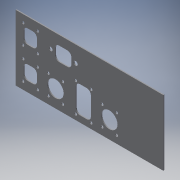
# Autodesk Inventor part: Plug-in Plate
Saved by Autodesk Inventor 2017 (Build 210142000, 142)
## iProperties
Created: 2017-03-05
Part Number: Plug-in Plate
Material: Generic
Document SubType Name: Modeling
Designer: coffmant
Density: 1 g/cm^3
Appearance: Default
Quantity: 1
Author: coffmant
Autodesk Inventor part; units mm, degrees
ref_plane "YZ Plane" through (0, 0, 0) normal (1, 0, 0) x (0, 1, 0)
ref_plane "XZ Plane" through (0, 0, 0) normal (0, 1, 0) x (-1, 0, 0)
ref_plane "XY Plane" through (0, 0, 0) normal (0, 0, 1) x (1, 0, 0)
sketch "Sketch1" plane through (0, 0, 0) normal (0, 0, 1) x (1, 0, 0)
  line L0 (0, 0) -> (228.6, 0)
  line L1 (228.6, 0) -> (228.6, -101.6)
  line L2 (228.6, -101.6) -> (0, -101.6)
  line L3 (0, -101.6) -> (0, 0)
  dimension "d0" = 101.6
  dimension "d1" = 228.6
  constraints: 8 end point, 2 parallel, 1 horizontal, 1 perpendicular
  measures "d0" distance of L2.end L0.start
  measures "d1" distance between parallel lines of L1 L3
extrude "Extrusion1" add sketch "Sketch1" along normal blind 1.5875
sketch "Sketch2" plane through (0, 0, 1.5875) normal (0, 0, 1) x (1, 0, 0)
  line L0 (18.3388, -37.6555) -> (26.6192, -37.6555)
  line L1 (32.9692, -31.3055) -> (32.9692, -21.9075)
  line L2 (26.6192, -15.5575) -> (18.3388, -15.5575)
  line L3 (11.9888, -21.9075) -> (11.9888, -31.3055)
  arc A0 (11.9888, -31.3055) -> (18.3388, -37.6555) centre (18.3388, -31.3055) ccw
  arc A1 (18.3388, -15.5575) -> (11.9888, -21.9075) centre (18.3388, -21.9075) ccw
  arc A2 (32.9692, -21.9075) -> (26.6192, -15.5575) centre (26.6192, -21.9075) ccw
  arc A3 (26.6192, -37.6555) -> (32.9692, -31.3055) centre (26.6192, -31.3055) ccw
  circle A4 centre (10.9982, -41.783) radius 2.1463
  circle A5 centre (33.7058, -11.43) radius 2.1463
  circle A6 centre (33.7058, -41.783) radius 2.1463
  circle A7 centre (11.2522, -11.43) radius 2.1463
  line L4 (6.35, -46.863) -> (38.1, -46.863)
  line L5 (38.1, -46.863) -> (38.1, -6.35)
  line L6 (38.1, -6.35) -> (6.35, -6.35)
  line L7 (6.35, -6.35) -> (6.35, -46.863)
  line L8 (228.6, 0) -> (0, 0) projected
  line L9 (0, 0) -> (0, -101.6) projected
  point P0 (32.9692, -15.5575)
  point P1 (32.9692, -37.6555)
  point P2 (11.9888, -15.5575)
  dimension "d4" = 20.9804
  dimension "d5" = 22.098
  dimension "d6" = 6.35
  dimension "d7" = 4.2926
  dimension "d8" = 4.2926
  dimension "d9" = 4.2926
  dimension "d10" = 4.2926
  dimension "d11" = 0.9906
  dimension "d12" = 0.7366
  dimension "d13" = 0.7366
  dimension "d14" = 0.7366
  dimension "d15" = 4.1275
  dimension "d16" = 4.1275
  dimension "d17" = 4.1275
  dimension "d18" = 4.1275
  dimension "d19" = 31.75
  dimension "d20" = 40.513
  dimension "d21" = 5.08
  dimension "d22" = 4.6482
  dimension "d26" = 6.35
  dimension "d27" = 6.35
  constraints: 16 end point, 8 centre point, 8 point on circle, 8 tangent, 6 point on line, 4 parallel, 3 equal radius, 2 horizontal, 2 perpendicular
  measures "d4" distance of point (11.989, -15.558) point (32.969, -15.558)
  measures "d5" distance of point (32.969, -15.558) point (32.969, -37.656)
  measures "d6" radius of A0
  measures "d7" diameter of A4
  measures "d8" diameter of A5
  measures "d9" diameter of A6
  measures "d10" diameter of A7
  measures "d11" distance from line of L3 A4.centre
  measures "d12" distance from line of L1 A6.centre
  measures "d13" distance from line of L1 A5.centre
  measures "d14" distance from line of A7.centre L3
  measures "d15" distance from line of L0 A4.centre
  measures "d16" distance from line of L0 A6.centre
  measures "d17" distance from line of L2 A5.centre
  measures "d18" distance from line of L2 A7.centre
  measures "d19" distance of L6.end L6.start
  measures "d20" distance of L6.start L5.start
  measures "d21" distance from line of A7.centre L6
  measures "d22" distance from line of L7 A4.centre
  measures "d26" distance between parallel lines of L8 L6
  measures "d27" distance between parallel lines of L7 L9
extrude "J9" cut sketch "Sketch2" against normal blind 1.5875 contours A0 L3 A1 L2 A2 L1 A3 L0 | A4 | A5 | A6 | A7
sketch "Sketch3" plane through (0, 0, 1.5875) normal (0, 0, 1) x (1, 0, 0)
  line L0 (67.183, -36.3982) -> (79.9084, -36.3982)
  line L1 (86.2584, -30.0482) -> (86.2584, -20.6502)
  line L2 (79.9084, -14.3002) -> (67.183, -14.3002)
  line L3 (60.833, -20.6502) -> (60.833, -30.0482)
  arc A0 (60.833, -30.0482) -> (67.183, -36.3982) centre (67.183, -30.0482) ccw
  arc A1 (79.9084, -36.3982) -> (86.2584, -30.0482) centre (79.9084, -30.0482) ccw
  arc A2 (86.2584, -20.6502) -> (79.9084, -14.3002) centre (79.9084, -20.6502) ccw
  arc A3 (67.183, -14.3002) -> (60.833, -20.6502) centre (67.183, -20.6502) ccw
  circle A4 centre (54.2417, -25.3492) radius 2.8067
  circle A5 centre (92.8497, -25.3492) radius 3.175
  line L4 (45.6692, -40.8432) -> (100.4062, -40.8432)
  line L5 (100.4062, -40.8432) -> (100.4062, -9.8552)
  line L6 (100.4062, -9.8552) -> (45.6692, -9.8552)
  line L7 (45.6692, -9.8552) -> (45.6692, -40.8432)
  line L8 (228.6, 0) -> (0, 0) projected
  line L9 (32.9692, -21.9075) -> (32.9692, -31.3055) projected
  dimension "d30" = 6.35
  dimension "d31" = 25.4254
  dimension "d32" = 22.098
  dimension "d33" = 5.6134
  dimension "d34" = 6.35
  dimension "d35" = 6.5913
  dimension "d36" = 6.5913
  dimension "d37" = 11.049
  dimension "d38" = 11.049
  dimension "d39" = 54.737
  dimension "d40" = 30.988
  dimension "d41" = 15.494
  dimension "d42" = 14.1478
  dimension "d98" = 12.7
  dimension "d99" = 9.8552
  constraints: 16 end point, 8 point on circle, 8 tangent, 6 centre point, 5 parallel, 3 equal radius, 2 perpendicular
  measures "d30" radius of A0
  measures "d31" distance between parallel lines of L1 L3
  measures "d32" distance between parallel lines of L2 L0
  measures "d33" diameter of A4
  measures "d34" diameter of A5
  measures "d35" distance from line of A4.centre L3
  measures "d36" distance from line of A5.centre L1
  measures "d37" distance from line of A4.centre L2
  measures "d38" distance from line of L2 A5.centre
  measures "d39" distance of L6.end L6.start
  measures "d40" distance of L6.start L4.end
  measures "d41" distance from line of A4.centre L6
  measures "d42" distance between parallel lines of L1 L5
  measures "d98" distance between parallel lines of L9 L7
  measures "d99" distance between parallel lines of L8 L6
extrude "J8" cut sketch "Sketch3" against normal blind 1.5875 contours A0 L3 A3 L2 A2 L1 A1 L0 | A4 | A5
sketch "Sketch4" plane through (0, 0, 1.5875) normal (0, 0, 1) x (1, 0, 0)
  circle A0 centre (61.5442, -74.9935) radius 12.7
  circle A1 centre (50.3174, -90.17) radius 2.159
  circle A2 centre (50.3174, -59.817) radius 2.159
  circle A3 centre (72.771, -90.17) radius 2.159
  circle A4 centre (72.771, -59.817) radius 2.159
  line L0 (45.6692, -95.25) -> (77.4192, -95.25)
  line L1 (77.4192, -95.25) -> (77.4192, -54.737)
  line L2 (77.4192, -54.737) -> (45.6692, -54.737)
  line L3 (45.6692, -54.737) -> (45.6692, -95.25)
  line L4 (228.6, 0) -> (0, 0) projected
  line L5 (0, 0) -> (0, -101.6) projected
  line L6 (0, -101.6) -> (228.6, -101.6) projected
  line L7 (32.9692, -21.9075) -> (32.9692, -31.3055) projected
  dimension "d49" = 25.4
  dimension "d50" = 4.318
  dimension "d51" = 4.318
  dimension "d52" = 4.318
  dimension "d53" = 4.318
  dimension "d54" = 11.2268
  dimension "d55" = 11.2268
  dimension "d56" = 11.2268
  dimension "d57" = 11.2268
  dimension "d58" = 15.1765
  dimension "d59" = 15.1765
  dimension "d60" = 15.1765
  dimension "d61" = 15.1765
  dimension "d62" = 31.75
  dimension "d63" = 40.513
  dimension "d64" = 5.08
  dimension "d65" = 4.6482
  dimension "d69" = 6.35
  dimension "d97" = 12.7
  constraints: 8 end point, 5 centre point, 2 parallel, 1 horizontal, 1 perpendicular
  measures "d49" diameter of A0
  measures "d50" diameter of A1
  measures "d51" diameter of A2
  measures "d52" diameter of A3
  measures "d53" diameter of A4
  measures "d54" horizontal distance of A0.centre A2.centre
  measures "d55" horizontal distance of A0.centre A1.centre
  measures "d56" horizontal distance of A0.centre A3.centre
  measures "d57" horizontal distance of A0.centre A4.centre
  measures "d58" vertical distance of A0.centre A2.centre
  measures "d59" vertical distance of A1.centre A0.centre
  measures "d60" vertical distance of A0.centre A3.centre
  measures "d61" vertical distance of A0.centre A4.centre
  measures "d62" distance of L1.end L2.end
  measures "d63" distance of L1.end L1.start
  measures "d64" distance from line of A2.centre L2
  measures "d65" distance from line of L3 A2.centre
  measures "d69" distance between parallel lines of L6 L0
  measures "d97" distance between parallel lines of L7 L3
extrude "J7" cut sketch "Sketch4" against normal blind 1.5875 contours A0 | A1 | A2 | A3 | A4
sketch "Sketch5" plane through (0, 0, 1.5875) normal (0, 0, 1) x (1, 0, 0)
  arc A0 (18.3388, -63.9445) -> (11.9888, -70.2945) centre (18.3388, -70.2945) ccw
  line L0 (32.9692, -79.6925) -> (32.9692, -70.2945)
  circle A1 centre (11.2522, -59.817) radius 2.1463
  line L1 (38.1, -54.737) -> (6.35, -54.737)
  line L2 (11.9888, -70.2945) -> (11.9888, -79.6925)
  line L3 (18.3388, -86.0425) -> (26.6192, -86.0425)
  line L4 (38.1, -95.25) -> (38.1, -54.737)
  line L5 (6.35, -54.737) -> (6.35, -95.25)
  line L6 (26.6192, -63.9445) -> (18.3388, -63.9445)
  circle A2 centre (33.7058, -59.817) radius 2.1463
  arc A3 (11.9888, -79.6925) -> (18.3388, -86.0425) centre (18.3388, -79.6925) ccw
  arc A4 (26.6192, -86.0425) -> (32.9692, -79.6925) centre (26.6192, -79.6925) ccw
  circle A5 centre (10.9982, -90.17) radius 2.1463
  circle A6 centre (33.7058, -90.17) radius 2.1463
  line L7 (6.35, -95.25) -> (38.1, -95.25)
  arc A7 (32.9692, -70.2945) -> (26.6192, -63.9445) centre (26.6192, -70.2945) ccw
  line L8 (228.6, 0) -> (0, 0)
  line L9 (0, 0) -> (0, -101.6)
  line L10 (0, -101.6) -> (228.6, -101.6) projected
  point P0 (11.9888, -63.9445)
  point P1 (32.9692, -63.9445)
  point P2 (32.9692, -86.0425)
  dimension "d72" = 20.9804
  dimension "d73" = 22.098
  dimension "d74" = 6.35
  dimension "d75" = 4.2926
  dimension "d76" = 4.2926
  dimension "d77" = 4.2926
  dimension "d78" = 4.2926
  dimension "d79" = 0.9906
  dimension "d80" = 0.7366
  dimension "d81" = 0.7366
  dimension "d82" = 0.7366
  dimension "d83" = 4.1275
  dimension "d84" = 4.1275
  dimension "d85" = 4.1275
  dimension "d86" = 4.1275
  dimension "d87" = 31.75
  dimension "d88" = 40.513
  dimension "d89" = 5.08
  dimension "d90" = 4.6482
  dimension "d93" = 6.35
  dimension "d94" = 6.35
  constraints: 20 end point, 8 centre point, 8 point on circle, 8 tangent, 6 point on line, 4 parallel, 3 equal radius, 2 horizontal, 2 perpendicular
  measures "d72" distance of point (11.989, -63.944) point (32.969, -63.944)
  measures "d73" distance of point (32.969, -63.944) point (32.969, -86.043)
  measures "d74" radius of A3
  measures "d75" diameter of A5
  measures "d76" diameter of A2
  measures "d77" diameter of A6
  measures "d78" diameter of A1
  measures "d79" distance from line of L2 A5.centre
  measures "d80" distance from line of L0 A6.centre
  measures "d81" distance from line of L0 A2.centre
  measures "d82" distance from line of A1.centre L2
  measures "d83" distance from line of L3 A5.centre
  measures "d84" distance from line of L3 A6.centre
  measures "d85" distance from line of L6 A2.centre
  measures "d86" distance from line of L6 A1.centre
  measures "d87" distance of L1.end L1.start
  measures "d88" distance of L1.start L4.start
  measures "d89" distance from line of A1.centre L1
  measures "d90" distance from line of L5 A5.centre
  measures "d93" distance between parallel lines of L10 L7
  measures "d94" distance between parallel lines of L9 L5
extrude "J6" cut sketch "Sketch5" against normal blind 1.5875 contours L6 A7 L0 A4 L3 A3 L2 A0 | A1 | A2 | A5 | A6
sketch "Sketch6" plane through (0, 0, 1.5875) normal (0, 0, 1) x (1, 0, 0)
  line L0 (99.314, -49.9491) -> (110.1344, -49.9491)
  line L1 (116.4844, -56.2991) -> (116.4844, -85.4329)
  line L2 (110.1344, -91.7829) -> (99.314, -91.7829)
  line L3 (92.964, -85.4329) -> (92.964, -56.2991)
  arc A0 (92.964, -85.4329) -> (99.314, -91.7829) centre (99.314, -85.4329) ccw
  arc A1 (110.1344, -91.7829) -> (116.4844, -85.4329) centre (110.1344, -85.4329) ccw
  arc A2 (116.4844, -56.2991) -> (110.1344, -49.9491) centre (110.1344, -56.2991) ccw
  arc A3 (99.314, -49.9491) -> (92.964, -56.2991) centre (99.314, -56.2991) ccw
  circle A4 centre (92.7862, -48.387) radius 2.1463
  circle A5 centre (116.6622, -48.387) radius 2.1463
  circle A6 centre (116.6622, -93.345) radius 2.1463
  circle A7 centre (92.7862, -93.345) radius 2.1463
  line L4 (86.9442, -98.425) -> (122.5042, -98.425)
  line L5 (122.5042, -98.425) -> (122.5042, -43.307)
  line L6 (122.5042, -43.307) -> (86.9442, -43.307)
  line L7 (86.9442, -43.307) -> (86.9442, -98.425)
  line L8 (228.6, 0) -> (0, 0) projected
  line L9 (0, -101.6) -> (228.6, -101.6) projected
  circle A8 centre (61.5442, -74.9935) radius 12.7 projected
  point P0 (92.964, -49.9491)
  point P1 (116.4844, -91.7829)
  point P2 (92.964, -91.7829)
  dimension "d100" = 23.5204
  dimension "d101" = 41.8338
  dimension "d102" = 6.35
  dimension "d103" = 0.1778
  dimension "d104" = 23.876
  dimension "d105" = 0.1778
  dimension "d106" = 1.5621
  dimension "d107" = 23.876
  dimension "d108" = 1.5621
  dimension "d109" = 1.5621
  dimension "d110" = 1.5621
  dimension "d111" = 35.56
  dimension "d112" = 55.118
  dimension "d113" = 5.08
  dimension "d114" = 5.842
  dimension "d115" = 4.2926
  dimension "d116" = 4.2926
  dimension "d117" = 4.2926
  dimension "d118" = 4.2926
  dimension "d121" = 3.175
  dimension "d122" = 12.7
  constraints: 16 end point, 8 centre point, 8 point on circle, 8 tangent, 6 point on line, 5 parallel, 3 equal radius, 2 perpendicular
  measures "d100" distance of point (116.484, -91.783) point (92.964, -91.783)
  measures "d101" distance of point (92.964, -49.949) point (92.964, -91.783)
  measures "d102" radius of A0
  measures "d103" distance from line of L3 A4.centre
  measures "d104" distance of A4.centre A5.centre
  measures "d105" distance from line of L3 A7.centre
  measures "d106" distance from line of A4.centre L0
  measures "d107" distance of A6.centre A7.centre
  measures "d108" distance from line of L0 A5.centre
  measures "d109" distance from line of L2 A7.centre
  measures "d110" distance from line of L2 A6.centre
  measures "d111" distance of L6.end L6.start
  measures "d112" distance of L6.end L4.start
  measures "d113" distance from line of A4.centre L6
  measures "d114" distance from line of L7 A4.centre
  measures "d115" diameter of A4
  measures "d116" diameter of A5
  measures "d117" diameter of A6
  measures "d118" diameter of A7
  measures "d121" distance between parallel lines of L4 L9
  measures "d122" distance edge to line of A8 L7
extrude "J11" cut sketch "Sketch6" against normal blind 1.5875 contours L0 A2 L1 A1 L2 A0 L3 A3 | A4 | A5 | A6 | A7
sketch "Sketch7" plane through (0, 0, 1.5875) normal (0, 0, 1) x (1, 0, 0)
  circle A0 centre (156.2862, -90.17) radius 2.159
  line L0 (160.9344, -95.25) -> (160.9344, -54.737)
  circle A1 centre (145.0594, -74.9935) radius 12.7
  circle A2 centre (133.8326, -59.817) radius 2.159
  line L1 (160.9344, -54.737) -> (129.1844, -54.737)
  line L2 (129.1844, -95.25) -> (160.9344, -95.25)
  circle A3 centre (156.2862, -59.817) radius 2.159
  circle A4 centre (133.8326, -90.17) radius 2.159
  line L3 (129.1844, -54.737) -> (129.1844, -95.25)
  line L4 (116.4844, -56.2991) -> (116.4844, -85.4329) projected
  line L5 (0, -101.6) -> (228.6, -101.6) projected
  point P0 (0, 0)
  dimension "d125" = 25.4
  dimension "d126" = 4.318
  dimension "d127" = 4.318
  dimension "d128" = 4.318
  dimension "d129" = 4.318
  dimension "d130" = 11.2268
  dimension "d131" = 11.2268
  dimension "d132" = 11.2268
  dimension "d133" = 11.2268
  dimension "d134" = 15.1765
  dimension "d135" = 15.1765
  dimension "d136" = 15.1765
  dimension "d137" = 15.1765
  dimension "d138" = 31.75
  dimension "d139" = 40.513
  dimension "d140" = 5.08
  dimension "d141" = 4.6482
  dimension "d144" = 12.7
  dimension "d146" = 6.35
  constraints: 8 end point, 5 centre point, 2 parallel, 1 horizontal, 1 perpendicular
  measures "d125" diameter of A1
  measures "d126" diameter of A4
  measures "d127" diameter of A2
  measures "d128" diameter of A0
  measures "d129" diameter of A3
  measures "d130" horizontal distance of A1.centre A2.centre
  measures "d131" horizontal distance of A1.centre A4.centre
  measures "d132" horizontal distance of A1.centre A0.centre
  measures "d133" horizontal distance of A1.centre A3.centre
  measures "d134" vertical distance of A1.centre A2.centre
  measures "d135" vertical distance of A4.centre A1.centre
  measures "d136" vertical distance of A1.centre A0.centre
  measures "d137" vertical distance of A1.centre A3.centre
  measures "d138" distance of L0.end L1.end
  measures "d139" distance of L0.end L0.start
  measures "d140" distance from line of A2.centre L1
  measures "d141" distance from line of L3 A2.centre
  measures "d144" distance between parallel lines of L3 L4
  measures "d146" distance between parallel lines of L5 L2
extrude "J4" cut sketch "Sketch7" against normal blind 1.5875 contours A0 | A1 | A2 | A3 | A4
equation "\"d27\" = d26"
equation "\"d37\" = 0.5 * d32"
equation "\"d41\" = 0.5 * d40"
equation "\"d94\" = d93"
body "Solid1"
